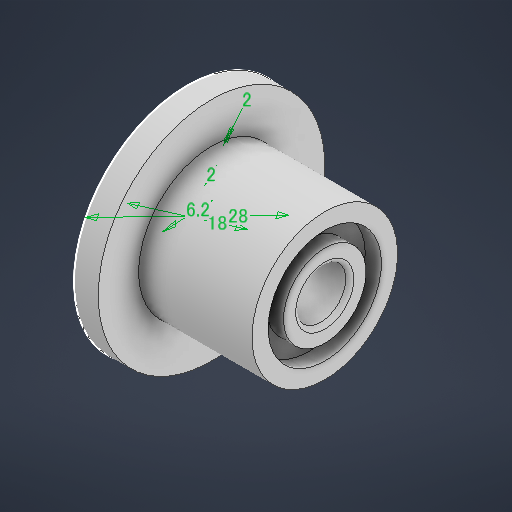
# Autodesk Inventor part: myPartbasic
Saved by Autodesk Inventor 2025.2 (Build 292293000, 293)
## iProperties
Created: 2024-11-22
Part Number: myPartbasic
Material: 一般
Document SubType Name: Modeling
Designer: ktamu
Density: 1 g/cm^3
Appearance: 既定
Author: ktamu
Autodesk Inventor part; units mm, degrees
ref_plane "YZ Plane" through (0, 0, 0) normal (1, 0, 0) x (0, 1, 0)
ref_plane "XZ Plane" through (0, 0, 0) normal (0, 1, 0) x (-1, 0, 0)
ref_plane "XY Plane" through (0, 0, 0) normal (0, 0, 1) x (1, 0, 0)
sketch "スケッチ1" plane through (0, 0, 0) normal (1, 0, 0) x (0, 1, 0)
  circle A0 centre (0, 0) radius 3.1
  circle A1 centre (0, 0) radius 9
  circle A2 centre (0, 0) radius 7
  circle A3 centre (0, 0) radius 5.1
  circle A4 centre (0, 0) radius 14
  dimension "d0" = 6.2
  dimension "d1" = 18
  dimension "d2" = 2
  dimension "d8" = 2
  dimension "d9" = 28
  constraints: 5 centre point, 5 coincident
  measures "d0" diameter of A0
  measures "d1" diameter of A1
  measures "d2" radial gap between concentric circles of A1 A2
  measures "d8" radial gap between concentric circles of A3 A0
  measures "d9" diameter of A4
extrude "押し出し1" add sketch "スケッチ1" along normal blind 17 contours A1 | A3
extrude "押し出し2" add sketch "スケッチ1" along normal blind 15 contours A2
fillet "フィレット1" radius 0.5 1 edges at (17, -3.1, 0)
extrude "押し出し3" add sketch "スケッチ1" along normal blind 3 contours A4
